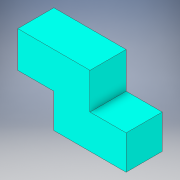
# Autodesk Inventor part: BluePiece
Saved by Autodesk Inventor 2019 (Build 230136000, 136)
## iProperties
Created: 2018-12-10
Part Number: BluePiece
Material: Generic
Document SubType Name: Modeling
Designer: Mihir
Density: 1 g/cm^3
Appearance: Default
Author: Mihir
Autodesk Inventor part; units mm, degrees
ref_plane "YZ Plane" through (0, 0, 0) normal (1, 0, 0) x (0, 1, 0)
ref_plane "XZ Plane" through (0, 0, 0) normal (0, 1, 0) x (-1, 0, 0)
ref_plane "XY Plane" through (0, 0, 0) normal (0, 0, 1) x (1, 0, 0)
sketch "Sketch1" plane through (0, 0, 0) normal (0, 0, 1) x (1, 0, 0)
  line L0 (0, 0) -> (38.1, 0)
  line L1 (38.1, 0) -> (38.1, 19.05)
  line L2 (38.1, 19.05) -> (0, 19.05)
  line L3 (0, 19.05) -> (0, 0)
  line L4 (19.05, 0) -> (57.15, 0)
  line L5 (57.15, 0) -> (57.15, -17.9755)
  line L6 (57.15, -17.9755) -> (19.05, -17.9755)
  line L7 (19.05, -17.9755) -> (19.05, 0)
  dimension "d0" = 38.1
  dimension "d1" = 19.05
  dimension "d2" = 19.05
  constraints: 16 end point, 4 parallel, 2 horizontal, 2 perpendicular, 1 midpoint
  measures "d0" distance of L1.end L2.end
  measures "d1" distance of L0.end L1.end
  measures "d2" distance of L0.end L4.end
extrude "Extrusion1" add sketch "Sketch1" along normal blind 19.05
body "Solid1"
